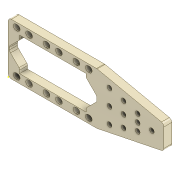
# Autodesk Inventor part: bracket_body_5mm
Saved by Autodesk Inventor 2020 (Build 240168000, 168)
## iProperties
Created: 2019-10-12
Part Number: bracket_body_5mm
Material: Generic
Document SubType Name: Modeling
Designer: WJ
Density: 1 g/cm^3
Appearance: Light Beige
Author: WJ
Autodesk Inventor part; units mm, degrees
ref_plane "YZ Plane" through (0, 0, 0) normal (1, 0, 0) x (0, 1, 0)
ref_plane "XZ Plane" through (0, 0, 0) normal (0, 1, 0) x (-1, 0, 0)
ref_plane "XY Plane" through (0, 0, 0) normal (0, 0, 1) x (1, 0, 0)
sketch "Sketch1" plane through (0, 0, 0) normal (0, 0, 1) x (1, 0, 0)
  line L0 (0, 0) -> (300, 0)
  line L1 (300, 0) -> (300, 33)
  line L2 (300, 33) -> (0, 33)
  line L3 (0, 33) -> (0, 0)
  dimension "d0" = 300
  dimension "d1" = 33
  constraints: 8 end point, 2 parallel, 1 horizontal, 1 perpendicular
  measures "d0" distance of L0.start L0.end
  measures "d1" distance of L2.end L0.start
extrude "Extrusion1" add sketch "Sketch1" along normal blind 5
sketch "Sketch3" plane through (0, 0, 0) normal (0, 0, -1) x (-1, 0, 0)
  arc A0 (-294.158, 28.337) -> (-294.158, 31.893) centre (-294.158, 30.115) ccw projected
  arc A1 (-294.92, 31.893) -> (-294.92, 28.337) centre (-294.92, 30.115) ccw projected
  arc A2 (-287.0308, 31.893) -> (-287.0308, 28.337) centre (-287.0308, 30.115) ccw projected
  arc A3 (-286.2688, 28.337) -> (-286.2688, 31.893) centre (-286.2688, 30.115) ccw projected
  arc A4 (-275.87, 31.893) -> (-275.87, 28.337) centre (-275.87, 30.115) ccw projected
  arc A5 (-275.108, 28.337) -> (-275.108, 31.893) centre (-275.108, 30.115) ccw projected
  arc A6 (-267.9808, 31.893) -> (-267.9808, 28.337) centre (-267.9808, 30.115) ccw projected
  arc A7 (-267.2188, 28.337) -> (-267.2188, 31.893) centre (-267.2188, 30.115) ccw projected
  arc A8 (-256.82, 31.893) -> (-256.82, 28.337) centre (-256.82, 30.115) ccw projected
  arc A9 (-256.058, 28.337) -> (-256.058, 31.893) centre (-256.058, 30.115) ccw projected
  arc A10 (-248.9308, 31.893) -> (-248.9308, 28.337) centre (-248.9308, 30.115) ccw projected
  arc A11 (-248.1688, 28.337) -> (-248.1688, 31.893) centre (-248.1688, 30.115) ccw projected
  circle A12 centre (-247.4017, 21.5976) radius 1.3525
  circle A13 centre (-247.4017, 11.6916) radius 1.3525
  arc A14 (-248.1688, 1.3962) -> (-248.1688, 4.9522) centre (-248.1688, 3.1742) ccw projected
  arc A15 (-248.9308, 4.9522) -> (-248.9308, 1.3962) centre (-248.9308, 3.1742) ccw projected
  arc A16 (-256.058, 1.3962) -> (-256.058, 4.9522) centre (-256.058, 3.1742) ccw projected
  arc A17 (-256.82, 4.9522) -> (-256.82, 1.3962) centre (-256.82, 3.1742) ccw projected
  arc A18 (-267.2188, 1.3962) -> (-267.2188, 4.9522) centre (-267.2188, 3.1742) ccw projected
  arc A19 (-267.9808, 4.9522) -> (-267.9808, 1.3962) centre (-267.9808, 3.1742) ccw projected
  arc A20 (-275.108, 1.3962) -> (-275.108, 4.9522) centre (-275.108, 3.1742) ccw projected
  arc A21 (-275.87, 4.9522) -> (-275.87, 1.3962) centre (-275.87, 3.1742) ccw projected
  arc A22 (-286.2688, 1.3962) -> (-286.2688, 4.9522) centre (-286.2688, 3.1742) ccw projected
  arc A23 (-287.0308, 4.9522) -> (-287.0308, 1.3962) centre (-287.0308, 3.1742) ccw projected
  arc A24 (-294.158, 1.3962) -> (-294.158, 4.9522) centre (-294.158, 3.1742) ccw projected
  arc A25 (-294.92, 4.9522) -> (-294.92, 1.3962) centre (-294.92, 3.1742) ccw projected
  arc A26 (-296.6, 8.8546) -> (-296.6, 13.7546) centre (-296.6, 11.3046) ccw
  arc A27 (-296.6, 18.8546) -> (-296.6, 23.7546) centre (-296.6, 21.3046) ccw
  arc A28 (-245.9, 23.7546) -> (-245.9, 18.8546) centre (-245.9, 21.3046) ccw
  arc A29 (-245.9, 13.7546) -> (-245.9, 8.8546) centre (-245.9, 11.3046) ccw
  arc A30 (-243.764, 12.5046) -> (-245.9, 13.7546) centre (-245.9, 11.3046) ccw
  arc A31 (-245.9, 8.8546) -> (-243.764, 10.1046) centre (-245.9, 11.3046) ccw
  arc A32 (-245.9, 18.8546) -> (-243.764, 20.1046) centre (-245.9, 21.3046) ccw
  arc A33 (-243.764, 22.5046) -> (-245.9, 23.7546) centre (-245.9, 21.3046) ccw
  arc A34 (-298.736, 20.1046) -> (-296.6, 18.8546) centre (-296.6, 21.3046) ccw
  arc A35 (-296.6, 23.7546) -> (-298.736, 22.5046) centre (-296.6, 21.3046) ccw
  arc A36 (-296.6, 13.7546) -> (-298.736, 12.5046) centre (-296.6, 11.3046) ccw
  arc A37 (-298.736, 10.1046) -> (-296.6, 8.8546) centre (-296.6, 11.3046) ccw
  line L0 (-294.92, 31.893) -> (-294.158, 31.893) projected
  line L1 (-294.158, 28.337) -> (-294.92, 28.337) projected
  line L2 (-286.2688, 28.337) -> (-287.0308, 28.337) projected
  line L3 (-287.0308, 31.893) -> (-286.2688, 31.893) projected
  line L4 (-275.108, 28.337) -> (-275.87, 28.337) projected
  line L5 (-275.87, 31.893) -> (-275.108, 31.893) projected
  line L6 (-267.9808, 31.893) -> (-267.2188, 31.893) projected
  line L7 (-267.2188, 28.337) -> (-267.9808, 28.337) projected
  line L8 (-248.9308, 31.893) -> (-248.1688, 31.893) projected
  line L9 (-248.1688, 28.337) -> (-248.9308, 28.337) projected
  line L10 (-256.058, 28.337) -> (-256.82, 28.337) projected
  line L11 (-256.82, 31.893) -> (-256.058, 31.893) projected
  line L12 (-248.9308, 4.9522) -> (-248.1688, 4.9522) projected
  line L13 (-248.1688, 1.3962) -> (-248.9308, 1.3962) projected
  line L14 (-256.058, 1.3962) -> (-256.82, 1.3962) projected
  line L15 (-256.82, 4.9522) -> (-256.058, 4.9522) projected
  line L16 (-267.9808, 4.9522) -> (-267.2188, 4.9522) projected
  line L17 (-267.2188, 1.3962) -> (-267.9808, 1.3962) projected
  line L18 (-275.87, 4.9522) -> (-275.108, 4.9522) projected
  line L19 (-275.108, 1.3962) -> (-275.87, 1.3962) projected
  line L20 (-287.0308, 4.9522) -> (-286.2688, 4.9522) projected
  line L21 (-286.2688, 1.3962) -> (-287.0308, 1.3962) projected
  line L22 (-294.158, 1.3962) -> (-294.92, 1.3962) projected
  line L23 (-294.92, 4.9522) -> (-294.158, 4.9522) projected
  circle A38 centre (-296.6, 21.3046) radius 2.5
  circle A39 centre (-296.6, 11.3046) radius 2.5
  circle A40 centre (-245.9, 21.3046) radius 2.5
  circle A41 centre (-245.9, 11.3046) radius 2.5
  line L24 (0, 0) -> (-300, 0) projected
  line L25 (-150, 0) -> (-150, 33) construction
  line L26 (-300, 33) -> (0, 33) projected
  arc A42 (-5.842, 31.893) -> (-5.842, 28.337) centre (-5.842, 30.115) ccw
  arc A43 (-5.08, 28.337) -> (-5.08, 31.893) centre (-5.08, 30.115) ccw
  arc A44 (-12.9692, 28.337) -> (-12.9692, 31.893) centre (-12.9692, 30.115) ccw
  arc A45 (-13.7312, 31.893) -> (-13.7312, 28.337) centre (-13.7312, 30.115) ccw
  arc A46 (-24.13, 28.337) -> (-24.13, 31.893) centre (-24.13, 30.115) ccw
  arc A47 (-24.892, 31.893) -> (-24.892, 28.337) centre (-24.892, 30.115) ccw
  arc A48 (-32.0192, 28.337) -> (-32.0192, 31.893) centre (-32.0192, 30.115) ccw
  arc A49 (-32.7812, 31.893) -> (-32.7812, 28.337) centre (-32.7812, 30.115) ccw
  arc A50 (-43.18, 28.337) -> (-43.18, 31.893) centre (-43.18, 30.115) ccw
  arc A51 (-43.942, 31.893) -> (-43.942, 28.337) centre (-43.942, 30.115) ccw
  arc A52 (-51.0692, 28.337) -> (-51.0692, 31.893) centre (-51.0692, 30.115) ccw
  arc A53 (-51.8312, 31.893) -> (-51.8312, 28.337) centre (-51.8312, 30.115) ccw
  circle A54 centre (-52.5983, 21.5976) radius 1.3525
  circle A55 centre (-52.5983, 11.6916) radius 1.3525
  arc A56 (-51.8312, 4.9522) -> (-51.8312, 1.3962) centre (-51.8312, 3.1742) ccw
  arc A57 (-51.0692, 1.3962) -> (-51.0692, 4.9522) centre (-51.0692, 3.1742) ccw
  arc A58 (-43.942, 4.9522) -> (-43.942, 1.3962) centre (-43.942, 3.1742) ccw
  arc A59 (-43.18, 1.3962) -> (-43.18, 4.9522) centre (-43.18, 3.1742) ccw
  arc A60 (-32.7812, 4.9522) -> (-32.7812, 1.3962) centre (-32.7812, 3.1742) ccw
  arc A61 (-32.0192, 1.3962) -> (-32.0192, 4.9522) centre (-32.0192, 3.1742) ccw
  arc A62 (-24.892, 4.9522) -> (-24.892, 1.3962) centre (-24.892, 3.1742) ccw
  arc A63 (-24.13, 1.3962) -> (-24.13, 4.9522) centre (-24.13, 3.1742) ccw
  arc A64 (-13.7312, 4.9522) -> (-13.7312, 1.3962) centre (-13.7312, 3.1742) ccw
  arc A65 (-12.9692, 1.3962) -> (-12.9692, 4.9522) centre (-12.9692, 3.1742) ccw
  arc A66 (-5.842, 4.9522) -> (-5.842, 1.3962) centre (-5.842, 3.1742) ccw
  arc A67 (-5.08, 1.3962) -> (-5.08, 4.9522) centre (-5.08, 3.1742) ccw
  arc A68 (-3.4, 13.7546) -> (-3.4, 8.8546) centre (-3.4, 11.3046) ccw
  arc A69 (-3.4, 23.7546) -> (-3.4, 18.8546) centre (-3.4, 21.3046) ccw
  arc A70 (-54.1, 18.8546) -> (-54.1, 23.7546) centre (-54.1, 21.3046) ccw
  arc A71 (-54.1, 8.8546) -> (-54.1, 13.7546) centre (-54.1, 11.3046) ccw
  arc A72 (-54.1, 13.7546) -> (-56.236, 12.5046) centre (-54.1, 11.3046) ccw
  arc A73 (-56.236, 10.1046) -> (-54.1, 8.8546) centre (-54.1, 11.3046) ccw
  arc A74 (-56.236, 20.1046) -> (-54.1, 18.8546) centre (-54.1, 21.3046) ccw
  arc A75 (-54.1, 23.7546) -> (-56.236, 22.5046) centre (-54.1, 21.3046) ccw
  arc A76 (-3.4, 18.8546) -> (-1.264, 20.1046) centre (-3.4, 21.3046) ccw
  arc A77 (-1.264, 22.5046) -> (-3.4, 23.7546) centre (-3.4, 21.3046) ccw
  arc A78 (-1.264, 12.5046) -> (-3.4, 13.7546) centre (-3.4, 11.3046) ccw
  arc A79 (-3.4, 8.8546) -> (-1.264, 10.1046) centre (-3.4, 11.3046) ccw
  line L27 (-5.08, 31.893) -> (-5.842, 31.893)
  line L28 (-5.842, 28.337) -> (-5.08, 28.337)
  line L29 (-13.7312, 28.337) -> (-12.9692, 28.337)
  line L30 (-12.9692, 31.893) -> (-13.7312, 31.893)
  line L31 (-24.892, 28.337) -> (-24.13, 28.337)
  line L32 (-24.13, 31.893) -> (-24.892, 31.893)
  line L33 (-32.0192, 31.893) -> (-32.7812, 31.893)
  line L34 (-32.7812, 28.337) -> (-32.0192, 28.337)
  line L35 (-51.0692, 31.893) -> (-51.8312, 31.893)
  line L36 (-51.8312, 28.337) -> (-51.0692, 28.337)
  line L37 (-43.942, 28.337) -> (-43.18, 28.337)
  line L38 (-43.18, 31.893) -> (-43.942, 31.893)
  line L39 (-51.0692, 4.9522) -> (-51.8312, 4.9522)
  line L40 (-51.8312, 1.3962) -> (-51.0692, 1.3962)
  line L41 (-43.942, 1.3962) -> (-43.18, 1.3962)
  line L42 (-43.18, 4.9522) -> (-43.942, 4.9522)
  line L43 (-32.0192, 4.9522) -> (-32.7812, 4.9522)
  line L44 (-32.7812, 1.3962) -> (-32.0192, 1.3962)
  line L45 (-24.13, 4.9522) -> (-24.892, 4.9522)
  line L46 (-24.892, 1.3962) -> (-24.13, 1.3962)
  line L47 (-12.9692, 4.9522) -> (-13.7312, 4.9522)
  line L48 (-13.7312, 1.3962) -> (-12.9692, 1.3962)
  line L49 (-5.842, 1.3962) -> (-5.08, 1.3962)
  line L50 (-5.08, 4.9522) -> (-5.842, 4.9522)
  circle A80 centre (-3.4, 21.3046) radius 2.5
  circle A81 centre (-3.4, 11.3046) radius 2.5
  circle A82 centre (-54.1, 21.3046) radius 2.5
  circle A83 centre (-54.1, 11.3046) radius 2.5
  line L51 (-300, 0) -> (0, 0)
  line L52 (0, 33) -> (-300, 33)
  point P0 (-52.3523, 13.0216)
  point P1 (-52.265, 13.0024)
  point P2 (-51.6729, 10.7052)
  point P3 (-51.7401, 10.6462)
  point P4 (-52.2429, 22.9026)
  point P5 (-52.1552, 22.8755)
  point P6 (-51.7073, 20.58)
  point P7 (-51.7784, 20.5219)
  point P8 (-248.2599, 10.6462)
  point P9 (-248.3271, 10.7052)
  point P10 (-247.735, 13.0024)
  point P11 (-247.6477, 13.0216)
  point P12 (-248.2216, 20.5219)
  point P13 (-248.2927, 20.58)
  point P14 (-247.8448, 22.8755)
  point P15 (-247.7571, 22.9026)
  dimension "d4" = 2.45
  dimension "d5" = 5
  dimension "d6" = 5
  dimension "d7" = 5
  dimension "d8" = 5
  constraints: 110 symmetric about line, 96 point on circle, 60 centre point, 54 end point, 8 coincident, 2 midpoint, 42 other
  measures "d4" radius of A33
  measures "d5" diameter of A40
  measures "d6" diameter of A41
  measures "d7" diameter of A38
  measures "d8" diameter of A39
extrude "Extrusion2" cut sketch "Sketch3" against normal mid plane 20 contours L1 A1 L0 A0 | L3 A3 L2 A2 | L5 A5 L4 A4 | L6 A7 L7 A6 | L11 A9 L10 A8 | L8 A11 L9 A10 | A12 A28 | A12 A40 | A13 A29 | A13 A41 | L13 A15 L12 A14 | L14 A17 L15 A16 | L17 A19 L16 A18 | L19 A21 L18 A20 | L21 A23 L20 A22 | L22 A25 L23 A24 | A39 | L27 A43 L28 A42 | L29 A45 L30 A44 | L31 A47 L32 A46 | L34 A49 L33 A48 | L37 A51 L38 A50 | L36 A53 L35 A52 | A54 A82 | A70 A54 | A55 A83 | A71 A55 | L39 A57 L40 A56 | L42 A59 L41 A58 | L43 A61 L44 A60 | L45 A63 L46 A62 | L47 A65 L48 A64 | L50 A67 L49 A66 | A80 | A81 picked at (-244.3082, 21.6054) picked at (-244.4141, 10.746) picked at (-55.6993, 21.2502) picked at (-55.5608, 10.6682)
sketch "Sketch4" plane through (0, 0, 0) normal (0, 0, -1) x (-1, 0, 0)
  line L0 (-292.709, 26.8899) -> (-250.301, 26.8899)
  line L1 (-250.301, 26.8899) -> (-250.301, 5.5886)
  line L2 (-250.301, 5.5886) -> (-292.709, 5.5886)
  line L3 (-292.709, 5.5886) -> (-292.709, 26.8899)
  line L4 (0, 0) -> (-300, 0) projected
  line L5 (-150, 0) -> (-150, 33) construction
  line L6 (-300, 33) -> (0, 33) projected
  line L7 (-7.291, 26.8899) -> (-49.699, 26.8899)
  line L8 (-49.699, 26.8899) -> (-49.699, 5.5886)
  line L9 (-49.699, 5.5886) -> (-7.291, 5.5886)
  line L10 (-7.291, 5.5886) -> (-7.291, 26.8899)
  constraints: 18 end point, 4 symmetric about line, 2 midpoint, 2 parallel, 1 horizontal, 1 perpendicular
extrude "Extrusion3" cut sketch "Sketch4" against normal mid plane 20
sketch "Sketch5" plane through (0, 0, 0) normal (0, 0, -1) x (-1, 0, 0)
  point P0 (0, 0)
sketch "Sketch7" plane through (0, 0, 0) normal (0, 0, -1) x (-1, 0, 0)
  arc A0 (-3.575, 13.8678) -> (-3.575, 18.7847) centre (-3.575, 16.3263) ccw
  line L0 (-3.575, 18.7847) -> (-7.2848, 18.7847)
  line L1 (-3.575, 13.8678) -> (-7.291, 13.8678)
  line L2 (-7.291, 26.8899) -> (-49.699, 26.8899) projected
  line L3 (-28.495, 26.8899) -> (-28.495, 5.5886) construction
  line L4 (-49.699, 5.5886) -> (-7.291, 5.5886) projected
  arc A1 (-53.415, 18.7847) -> (-53.415, 13.8678) centre (-53.415, 16.3263) ccw
  line L5 (-53.415, 18.7847) -> (-49.7052, 18.7847)
  line L6 (-53.415, 13.8678) -> (-49.699, 13.8678)
  line L7 (-49.7052, 18.7847) -> (-48.7948, 18.7847)
  line L8 (-48.7948, 18.7847) -> (-7.2848, 18.7847)
  line L9 (-7.291, 13.8678) -> (-49.699, 13.8678)
  line L10 (-7.291, 5.5886) -> (-7.291, 26.8899) projected
  point P0 (0, 0)
  constraints: 16 end point, 5 symmetric about line, 4 point on circle, 2 centre point, 2 midpoint, 2 tangent, 1 collinear, 1 horizontal, 1 perpendicular, 1 other
extrude "Extrusion5" cut sketch "Sketch7" against normal blind 10
sketch "Sketch8" plane through (0, 0, 0) normal (0, 0, -1) x (-1, 0, 0)
  line L0 (-300, 33) -> (0, 33) projected
  line L1 (-150, 33) -> (-150, 0) construction
  line L2 (0, 0) -> (-300, 0) projected
  line L3 (-53.4111, 18.8319) -> (-49.2836, 18.8319) projected
  arc A0 (-53.4111, 18.8319) -> (-53.4111, 13.8789) centre (-53.4111, 16.3554) ccw projected
  line L4 (-49.2836, 13.8789) -> (-53.4111, 13.8789) projected
  line L5 (-7.6276, 18.8319) -> (-3.5001, 18.8319) projected
  arc A1 (-3.5001, 13.8789) -> (-3.5001, 18.8319) centre (-3.5001, 16.3554) ccw projected
  line L6 (-3.5001, 13.8789) -> (-7.6276, 13.8789) projected
  line L7 (-246.5889, 18.8319) -> (-250.7164, 18.8319)
  arc A2 (-246.5889, 13.8789) -> (-246.5889, 18.8319) centre (-246.5889, 16.3554) ccw
  line L8 (-250.7164, 13.8789) -> (-246.5889, 13.8789)
  line L9 (-292.3724, 18.8319) -> (-296.4999, 18.8319)
  arc A3 (-296.4999, 18.8319) -> (-296.4999, 13.8789) centre (-296.4999, 16.3554) ccw
  line L10 (-296.4999, 13.8789) -> (-292.3724, 13.8789)
  line L11 (-292.3724, 18.8319) -> (-250.7164, 18.8319)
  line L12 (-250.301, 5.5886) -> (-250.301, 26.8899) projected
  line L13 (-250.7164, 13.8789) -> (-292.3724, 13.8789)
  line L14 (-292.709, 26.8899) -> (-292.709, 5.5886) projected
  point P0 (-298, 33)
  point P1 (-2, 33)
  point P2 (-2, 0)
  point P3 (-298, 0)
  constraints: 14 end point, 11 symmetric about line, 4 point on circle, 2 centre point, 2 midpoint, 2 perpendicular, 2 other
extrude "Extrusion6" cut sketch "Sketch8" against normal blind 10
sketch "Sketch9" plane through (0, 0, 5) normal (0, 0, 1) x (1, 0, 0)
  point P0 (0, 0)
sketch "Sketch10" plane through (0, 0, 5) normal (0, 0, 1) x (1, 0, 0)
  line L0 (0.9, 23.8046) -> (56.6043, 23.8046)
  line L1 (56.6043, 23.8046) -> (56.6043, 8.7282)
  line L2 (56.6043, 8.7282) -> (0.9, 8.7282)
  line L3 (0.9, 8.7282) -> (0.9, 23.8046)
  circle A0 centre (64.699, 16.2664) radius 1.5
  circle A1 centre (73.699, 16.2664) radius 1.5
  circle A2 centre (82.699, 16.2664) radius 1.5
  line L4 (49.699, 26.8899) -> (49.699, 18.7847) projected
  line L5 (99.4128, 16.2664) -> (99.4128, 23.8046)
  line L6 (99.4128, 23.8046) -> (56.6043, 33)
  line L7 (300, 33) -> (0, 33) projected
  line L8 (99.4128, 16.2664) -> (99.4128, 8.7282)
  line L9 (99.4128, 8.7282) -> (56.6043, 0)
  line L10 (0, 0) -> (300, 0) projected
  line L11 (56.6043, 0) -> (300.3248, -0.1651)
  line L12 (300.3248, -0.1651) -> (300.3488, 35.2466)
  line L13 (300.3488, 35.2466) -> (56.6043, 33)
  point P0 (298, 33)
  point P1 (2, 33)
  point P2 (2, 0)
  point P3 (298, 0)
  dimension "d27" = 15
  dimension "d28" = 3
  dimension "d29" = 9
  dimension "d30" = 3
  dimension "d31" = 9
  dimension "d32" = 3
  constraints: 22 end point, 3 centre point, 3 point on line, 2 parallel, 2 perpendicular, 1 horizontal, 1 vertical
  measures "d27" distance from line of A0.centre L4
  measures "d28" diameter of A0
  measures "d29" distance of A1.centre A0.centre
  measures "d30" diameter of A1
  measures "d31" distance of A2.centre A1.centre
  measures "d32" diameter of A2
extrude "Extrusion7" cut sketch "Sketch10" against normal blind 10
sketch "Sketch11" plane through (0, 0, 5) normal (0, 0, 1) x (1, 0, 0)
  arc A0 (51.8312, 28.337) -> (51.8312, 31.893) centre (51.8312, 30.115) ccw projected
  line L0 (51.8312, 30.115) -> (99.4128, 16.2664) construction
  line L1 (99.4128, 23.8046) -> (99.4128, 8.7282) projected
  circle A1 centre (64.699, 26.3699) radius 1.5
  circle A2 centre (73.699, 23.7504) radius 1.5
  circle A3 centre (82.699, 21.131) radius 1.5
  circle A4 centre (91.699, 16.2664) radius 1.5
  line L2 (99.4128, 16.2664) -> (95.6773, 16.2664) construction
  circle A5 centre (64.699, 6.163) radius 1.5
  circle A6 centre (73.699, 8.7824) radius 1.5
  circle A7 centre (82.699, 11.4019) radius 1.5
  point P0 (0, 0)
  dimension "d35" = 3
  dimension "d36" = 3
  dimension "d37" = 3
  dimension "d38" = 3
  dimension "d39" = 9
  constraints: 7 centre point, 4 end point, 3 point on line, 3 symmetric about line, 1 horizontal, 1 midpoint, 3 other
  measures "d35" diameter of A1
  measures "d36" diameter of A2
  measures "d37" diameter of A3
  measures "d38" diameter of A4
  measures "d39" horizontal distance of A3.centre A4.centre
extrude "Extrusion8" cut sketch "Sketch11" against normal blind 10
fillet "Fillet2" radius 2 2 edges at (99.4128, 23.8046, 2.5) (99.4128, 8.7282, 2.5)
chamfer "Chamfer1" distance 6 angle 45 4 edges at (0.9, 23.8046, 2.5) (0.9, 8.7282, 2.5) (56.6043, 23.8046, 2.5) (56.6043, 8.7282, 2.5)
fillet "Fillet5" radius 2 9 edges at (56.6043, 33, 2.5) (7.291, 23.8046, 2.5) (49.699, 23.8046, 2.5) (7.291, 8.7282, 2.5) (49.699, 8.7282, 2.5) (0.9, 17.8046, 2.5) (0.9, 14.7282, 2.5) (56.6043, 14.7282, 2.5) (56.6043, 17.8046, 2.5)
fillet "Fillet6" radius 2 2 edges at (0, 33, 2.5) (0, 0, 2.5)
body "Solid1"
